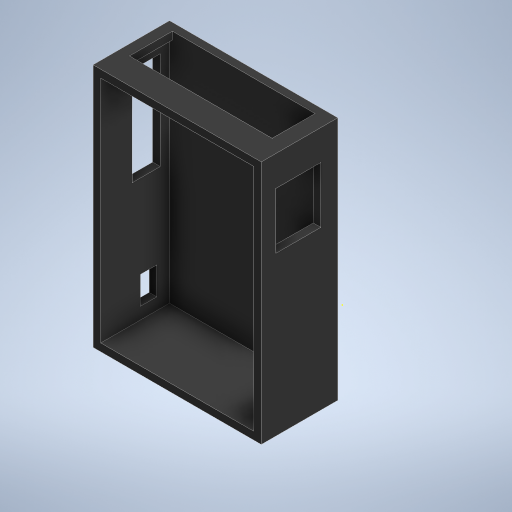
# Autodesk Inventor part: Part1
Saved by Autodesk Inventor 2023 (Build 270158000, 158)
## iProperties
Created: 2024-05-16
Part Number: Part1
Material: Rubber
Document SubType Name: Modeling
Designer: PRE 7730
Density: 0.93 g/cm^3
Appearance: Rubber - Black
Author: PRE 7730
Autodesk Inventor part; units mm, degrees
ref_plane "YZ Plane" through (0, 0, 0) normal (1, 0, 0) x (0, 1, 0)
ref_plane "XZ Plane" through (0, 0, 0) normal (0, 1, 0) x (-1, 0, 0)
ref_plane "XY Plane" through (0, 0, 0) normal (0, 0, 1) x (1, 0, 0)
sketch "Sketch3" plane through (0, 0, 0) normal (0, 0, 1) x (1, 0, 0)
  line L0 (-163.0852, 54.3849) -> (-53.0852, 54.3849)
  line L1 (-53.0852, 54.3849) -> (-53.0852, -105.6151)
  line L2 (-53.0852, -105.6151) -> (-163.0852, -105.6151)
  line L3 (-163.0852, -105.6151) -> (-163.0852, 54.3849)
  point P0 (0, 0)
  dimension "d2" = 110
  dimension "d3" = 160
  dimension "d4" = 110
  constraints: 8 end point, 2 perpendicular, 1 horizontal
  measures "d2" distance of L0.start L0.end
  measures "d3" distance of L0.end L1.end
  measures "d4" distance of L1.end L2.end
extrude "Extrusion1" add sketch "Sketch3" along normal blind 50
sketch "Sketch4" plane through (0, 0, 50) normal (0, 0, 1) x (1, 0, 0)
  point P0 (0, 0)
sketch "Sketch5" plane through (0, 0, 50) normal (0, 0, 1) x (1, 0, 0)
  line L0 (-163.0852, 54.3849) -> (-163.0852, -105.6151) projected
  line L1 (-163.0852, 54.3849) -> (-163.0852, 49.3849)
  line L2 (-163.0852, 49.3849) -> (-158.0852, 49.3849)
  line L3 (-158.0852, 49.3849) -> (-158.0852, -100.6151)
  line L4 (-158.0852, -100.6151) -> (-58.0852, -100.6151)
  line L5 (-58.0852, -100.6151) -> (-58.0852, 49.3849)
  line L6 (-58.0852, 49.3849) -> (-158.0852, 49.3849)
  point P0 (0, 0)
  dimension "d7" = 5
  dimension "d8" = 5
  dimension "d9" = 150
  dimension "d10" = 100
  constraints: 12 end point, 3 perpendicular, 1 horizontal, 1 point on line, 1 vertical
  measures "d7" distance of L0.start L1.end
  measures "d8" distance of L1.end L2.end
  measures "d9" distance of L2.end L3.end
  measures "d10" distance of L3.end L4.end
extrude "Extrusion2" cut sketch "Sketch5" against normal blind 45
sketch "Sketch6" plane through (-163.0852, 54.3849, 0) normal (0, 1, 0) x (1, 0, 0)
  line L0 (5, -5) -> (105, -5) projected
  line L1 (100.1792, -33.0786) -> (6.8805, -33.0786)
  line L2 (6.8805, -33.0786) -> (6.8805, -5)
  line L3 (6.8805, -5) -> (100.1792, -5)
  line L4 (100.1792, -5) -> (100.1792, -33.0786)
  point P0 (163.0852, 0)
  constraints: 8 end point, 2 parallel, 1 horizontal, 1 perpendicular, 1 point on line
extrude "Extrusion3" cut sketch "Sketch6" against normal blind 45
sketch "Sketch7" plane through (-163.0852, -105.6151, 0) normal (-1, 0, 0) x (0, 0, 1)
  line L0 (29.4052, 149.2988) -> (11.027, 149.2988)
  line L1 (11.027, 149.2988) -> (11.027, 85.399)
  line L2 (11.027, 85.399) -> (29.4052, 85.399)
  line L3 (29.4052, 85.399) -> (29.4052, 149.2988)
  line L4 (24.0331, 12.7342) -> (13.2889, 12.7342)
  line L5 (13.2889, 12.7342) -> (13.2889, 30.8297)
  line L6 (13.2889, 30.8297) -> (24.0331, 30.8297)
  line L7 (24.0331, 30.8297) -> (24.0331, 12.7342)
  point P0 (0, 105.6151)
  constraints: 16 end point, 4 parallel, 2 horizontal, 2 perpendicular
extrude "Extrusion4" cut sketch "Sketch7" against normal blind 45 contours L3 L2 L1 L0
extrude "Extrusion5" cut sketch "Sketch7" against normal blind 45 contours L4 L5 L6 L7
sketch "Sketch8" plane through (-58.0852, -100.6151, 50) normal (-1, 0, 0) x (0, 0, 1)
  line L0 (-38.973, 144.2988) -> (-38.973, 80.399) projected
  line L1 (-9.5905, 135.2241) -> (-38.973, 135.2241)
  line L2 (-38.973, 135.2241) -> (-38.973, 98.4676)
  line L3 (-38.973, 98.4676) -> (-9.5905, 98.4676)
  line L4 (-9.5905, 98.4676) -> (-9.5905, 135.2241)
  point P0 (-50, 100.6151)
  constraints: 8 end point, 2 parallel, 1 horizontal, 1 perpendicular, 1 point on line
extrude "Extrusion6" cut sketch "Sketch8" against normal blind 45
body "Solid1"
